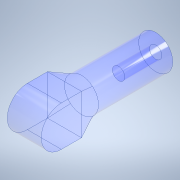
# Autodesk Inventor part: shank_2
Saved by Autodesk Inventor 2020.2 (Build 242310000, 310)
## iProperties
Created: 2021-01-30
Part Number: shank_2
Material: Generic
Document SubType Name: Modeling
Designer: DELL
Density: 1 g/cm^3
Appearance: Clear - Blue
Author: DELL
Autodesk Inventor part; units mm, degrees
ref_plane "YZ Plane" through (0, 0, 0) normal (1, 0, 0) x (0, 1, 0)
ref_plane "XZ Plane" through (0, 0, 0) normal (0, 1, 0) x (-1, 0, 0)
ref_plane "UCS1: YZ Plane" through (0, 0, 0) normal (1, 0, 0) x (0, 1, 0)
sketch "Sketch6" plane through (0, 0, 0) normal (1, 0, 0) x (0, 1, 0)
  circle A0 centre (0, 0) radius 32.5
  line L0 (-32.5, 0) -> (-32.5, -60)
  line L1 (-32.5, -60) -> (32.5, -60)
  line L2 (32.5, -60) -> (32.5, 0)
  line L3 (0, 0) -> (0, -60) construction
  line L4 (-32.5, -32.5) -> (32.5, -32.5)
  dimension "d38" = 65
  dimension "d39" = 60
  constraints: 10 end point, 3 perpendicular, 2 point on circle, 2 point on line, 2 tangent, 2 vertical, 1 centre point, 1 coincident, 1 midpoint
  measures "d38" diameter of A0
  measures "d39" distance from line of L1 point (0, 0)
extrude "Extrusion8" add sketch "Sketch6" along normal mid plane 55 contours A0 | L2 L4 A0 | A0 L4 L0
ref_plane "Work Plane2" through (0, -32.5, -60) normal (0, 0, -1) x (0, 1, 0)
ref_plane "Work Plane1" through (0, 0, 27.5) normal (0, 0, 1) x (1, 0, 0)
sketch "Sketch3" plane through (0, -32.5, -60) normal (0, 0, -1) x (0, 1, 0)
  circle A0 centre (32.5, 0) radius 27.5
  line L0 (65, -27.5) -> (65, 27.5) projected
  circle A1 centre (32.5, 0) radius 37.5
  dimension "d48" = 10
  dimension "d73" = 55
  constraints: 2 centre point, 2 coincident
  measures "d48" radial gap between concentric circles of A0 A1
  measures "d73" diameter of A0
loft "Loft1" add profiles "Sketch3" section 1 edges at (0, 32.5, -32.5) (27.5, 0, -32.5) (0, -32.5, -32.5) (-27.5, 0, -32.5) contours A0
sketch "Sketch7" plane through (0, 0, 0) normal (1, 0, 0) x (0, 1, 0)
  line L0 (20.9931, -60) -> (-20.9931, -60) projected
  line L1 (0, -60) -> (0, -180)
  point P0 (0, 0)
  dimension "d52" = 120
  constraints: 2 end point, 1 midpoint, 1 vertical
  measures "d52" distance from line of L0 L1.end
ref_plane "Work Plane3" through (0, 0, -180) normal (0, 0, -1) x (-1, 0, 0)
extrude "Extrusion1" add sketch "Sketch3" along normal blind 120 contours A0
sketch "Sketch5" plane through (0, 0, -180) normal (0, 0, -1) x (-1, 0, 0)
  circle A0 centre (0, 0) radius 10
  point P0 (0, 0)
  dimension "d35" = 20
  constraints: 1 centre point, 1 coincident
  measures "d35" diameter of A0
extrude "Extrusion7" cut sketch "Sketch5" against normal blind 60
body "Solid1"
body "Solid4"
